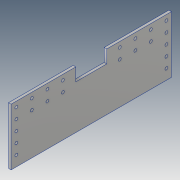
# Autodesk Inventor part: 200-40-BOGIE-CONNECTOR-06
Saved by Autodesk Inventor 2018.2 (Build 222227000, 227)
## iProperties
Manager: feesmrt
Company: FRANCOR
Part Number: 200-40-BOGIE-CONNECTOR-06
Project: Rescue Robot
Cost Center: -
Material: Aluminium 6061
Document SubType Name: Modeling
Designer: feesmrt
Engineer: feesmrt
Authority: feesmrt
Density: 2.7 g/cm^3
Appearance: Aluminium - flach
Description: Bogie Connector Verstärkungsplatte
Stock Number: 200-40-BOGIE-CONNECTOR-06
Mass: 165.052 g
Surface Area: 105.648 cm^2
Volume: 20.6315 cm^3
Subject: Rescue Robot
Author: feesmrt
Revision Number: 1
Title: Bogie Connector Verstärkungsplatte
Autodesk Inventor part; units mm, degrees
ref_plane "YZ Plane" through (0, 0, 0) normal (1, 0, 0) x (0, 1, 0)
ref_plane "XZ Plane" through (0, 0, 0) normal (0, 1, 0) x (-1, 0, 0)
ref_plane "XY Plane" through (0, 0, 0) normal (0, 0, 1) x (1, 0, 0)
sketch "Skizze1" plane through (0, 0, 0) normal (1, 0, 0) x (0, 1, 0)
  line L0 (-155, -55) -> (155, -55)
  line L1 (155, -55) -> (155, 55)
  line L2 (155, 55) -> (-155, 55)
  line L3 (-155, 55) -> (-155, -55)
  line L4 (-155, -55) -> (155, 55) construction
  line L5 (155, -55) -> (-155, 55) construction
  point P0 (0, 0)
  dimension "d43" = 310
  dimension "d44" = 110
  constraints: 12 end point, 2 midpoint, 2 parallel, 1 horizontal, 1 perpendicular
  measures "d43" distance of L1.end L2.end
  measures "d44" distance of L0.end L1.end
extrude "Grundlörper" add sketch "Skizze1" along normal blind 5
sketch "Skizze5" plane through (5, 0, 0) normal (1, 0, 0) x (0, 0, -1)
  line L0 (-55, -155) -> (55, -155) construction
  line L1 (-55, 155) -> (-55, -155) construction
  line L2 (55, 155) -> (-55, 155) construction
  line L3 (-91, 0) -> (91, 0) construction
  line L4 (0, -217) -> (0, 217) construction
  line L5 (-55, -30) -> (-30, -30)
  line L6 (-30, -30) -> (-30, 30)
  line L7 (-30, 30) -> (-55, 30)
  line L8 (-55, -30) -> (-55, 30)
  point P0 (0, 0)
  dimension "d50" = 60
  dimension "d51" = 25
  constraints: 8 end point, 2 point on line, 2 vertical, 1 perpendicular, 1 other
  measures "d50" distance between parallel lines of L7 L5
  measures "d51" distance of L5.start L5.end
extrude "Aussschnitt" cut sketch "Skizze5" against normal through all
sketch "Skizze7" plane through (5, 0, 0) normal (1, 0, 0) x (0, 0, -1)
  line L0 (-77, 0) -> (77, 0) projected
  line L1 (-55, -145) -> (55, -145) construction
  line L2 (55, -155) -> (55, 155) construction
  line L3 (-55, -155) -> (55, -155) construction
  line L4 (-55, -30) -> (-55, -155) construction
  line L5 (-55, 145) -> (55, 145) construction
  point P0 (0, 0)
  point P1 (-45, -145)
  point P2 (-25, -145)
  point P3 (-5, -145)
  point P4 (15, -145)
  point P5 (35, -145)
  point P6 (-45, -115)
  point P7 (-45, -85)
  point P8 (-45, -55)
  point P9 (-25, -145)
  point P10 (-25, -115)
  point P11 (-25, -85)
  point P12 (-25, -55)
  point P13 (-45, 145)
  point P14 (-25, 145)
  point P15 (-5, 145)
  point P16 (15, 145)
  point P17 (35, 145)
  point P18 (-45, 115)
  point P19 (-45, 85)
  point P20 (-45, 55)
  point P21 (-25, 145)
  point P22 (-25, 115)
  point P23 (-25, 85)
  point P24 (-25, 55)
  dimension "d104" = 10
  dimension "d105" = 10
  dimension "d108" = 20
  dimension "d115" = 30
  dimension "d118" = 20
  constraints: 14 symmetric about line, 4 end point, 4 point on line, 3 horizontal, 1 vertical, 11 other
  measures "d104" distance between parallel lines of L3 L1
  measures "d105" distance from line of L4 point (-45, -145)
  measures "d108" distance of point (-45, -145) point (-25, -145)
  measures "d115" distance of point (-45, -145) point (-45, -115)
  measures "d118" distance of point (-45, -145) point (-25, -145)
hole "Bohrung4" at (5, -145, 45) at (5, -145, 25) at (5, -145, 5) at (5, -145, -15) at (5, -145, -35) at (5, -115, 45) at (5, -85, 45) at (5, -55, 45) at (5, -115, 25) at (5, -85, 25) at (5, -55, 25) at (5, 55, 25) at (5, 85, 25) at (5, 115, 25) at (5, 145, 25) at (5, 55, 45) at (5, 85, 45) at (5, 115, 45) at (5, 145, -35) at (5, 145, -15) at (5, 145, 5) at (5, 145, 45) direction (-1, 0, 0) diameter 5.5 end through all
